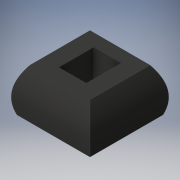
# Autodesk Inventor part: keyswitch-base_cherrymx
Saved by Autodesk Inventor 2016 (Build 200138000, 138)
## iProperties
Created: 2016-12-08
Part Number: keyswitch-base_cherrymx
Material: Generic
Document SubType Name: Modeling
Designer: Cemra JC
Density: 1 g/cm^3
Appearance: Default
Author: Cemra JC
Autodesk Inventor part; units mm, degrees
ref_plane "YZ Plane" through (0, 0, 0) normal (1, 0, 0) x (0, 1, 0)
ref_plane "XZ Plane" through (0, 0, 0) normal (0, 1, 0) x (-1, 0, 0)
ref_plane "XY Plane" through (0, 0, 0) normal (0, 0, 1) x (1, 0, 0)
sketch "Base Loop" plane through (0, 0, 0) normal (0, 1, 0) x (-1, 0, 0)
  line L0 (-7.3, 7.3) -> (7.3, 7.3)
  line L1 (7.3, 7.3) -> (7.3, -7.3)
  line L2 (7.3, -7.3) -> (-7.3, -7.3)
  line L3 (-7.3, -7.3) -> (-7.3, 7.3)
  line L4 (-7.3, 7.3) -> (7.3, -7.3) construction
  line L5 (7.3, 7.3) -> (-7.3, -7.3) construction
  point P0 (0, 0)
  point P1 (0, 0)
  point P2 (0, 0)
  dimension "d0" = 14.6
  dimension "d1" = 14.6
  constraints: 12 end point, 3 midpoint, 2 parallel, 1 coincident, 1 horizontal, 1 perpendicular
  measures "d0" distance of L1.end L2.end
  measures "d1" distance of L0.end L1.end
ref_plane "Mid Plane" through (-7.3, 2, -7.3) normal (0, 1, 0) x (1, 0, 0)
ref_plane "Base Plane" through (-7.3, 0, -7.3) normal (0, 1, 0) x (1, 0, 0)
sketch "Mid Loop" plane through (-7.3, 2, -7.3) normal (0, 1, 0) x (1, 0, 0)
  line L0 (14.5, -14.5) -> (0.1, -14.5)
  line L1 (0.1, -14.5) -> (0.1, -0.1)
  line L2 (0.1, -0.1) -> (14.5, -0.1)
  line L3 (14.5, -0.1) -> (14.5, -14.5)
  line L4 (14.5, -14.5) -> (0.1, -0.1) construction
  line L5 (0.1, -14.5) -> (14.5, -0.1) construction
  point P0 (7.3, -7.3)
  dimension "d3" = 14.4
  dimension "d4" = 14.4
  constraints: 12 end point, 2 midpoint, 2 parallel, 1 horizontal, 1 perpendicular
  measures "d3" distance of L0.end L1.end
  measures "d4" distance of L1.end L2.end
ref_plane "Top Plane" through (-7.3, 8.6, -7.3) normal (0, 1, 0) x (1, 0, 0)
sketch "Top Loop" plane through (-7.3, 8.6, -7.3) normal (0, 1, 0) x (1, 0, 0)
  line L0 (13.3, -13.3) -> (1.3, -13.3)
  line L1 (1.3, -13.3) -> (1.3, -1.3)
  line L2 (1.3, -1.3) -> (13.3, -1.3)
  line L3 (13.3, -1.3) -> (13.3, -13.3)
  line L4 (13.3, -13.3) -> (1.3, -1.3) construction
  line L5 (1.3, -13.3) -> (13.3, -1.3) construction
  point P0 (7.3, -7.3)
  dimension "d6" = 12
  dimension "d7" = 12
  constraints: 12 end point, 2 midpoint, 2 parallel, 1 horizontal, 1 perpendicular
  measures "d6" distance of L1.end L2.end
  measures "d7" distance of L0.end L1.end
loft "Keyswitch Body" add profiles "Base Loop", "Mid Loop", "Top Loop"
sketch "Cut in profile" plane through (-6, 8.6, 6) normal (0, 1, 0) x (1, 0, 0)
  line L0 (8.7, 2.275) -> (3.3, 2.275)
  line L1 (3.3, 2.275) -> (3.3, 9.725)
  line L2 (3.3, 9.725) -> (8.7, 9.725)
  line L3 (8.7, 9.725) -> (8.7, 2.275)
  line L4 (8.7, 2.275) -> (3.3, 9.725) construction
  line L5 (3.3, 2.275) -> (8.7, 9.725) construction
  point P0 (6, 6)
  dimension "d17" = 7.45
  dimension "d18" = 5.4
  constraints: 12 end point, 2 midpoint, 2 parallel, 1 horizontal, 1 perpendicular
  measures "d17" distance of L0.end L1.end
  measures "d18" distance of L0.start L0.end
extrude "Pole Cut in" cut sketch "Cut in profile" against normal blind 6.6
equation "\"d1\" = d0"
equation "\"d3\" = s_bwidth"
equation "\"d4\" = d3"
equation "\"d17\" = s_polebl"
equation "\"d18\" = s_polebw"
equation "\"k_width\" = 18.2"
equation "\"k_height\" = 16.5"
equation "\"k_taper1\" = 1.5"
equation "\"k_taper2\" = 0.5"
equation "\"k_radius\" = 6"
equation "\"k_wthick\" = 1.5"
equation "\"k_ribthick\" = 1.5"
equation "\"k_ribheight\" = 5"
equation "\"k_poleoff\" = 2.275"
equation "\"k_poledia\" = 5.3"
equation "\"k_cmxw\" = 1.55"
equation "\"k_cmxl\" = 4.35"
equation "\"s_bwidth\" = 14.4"
equation "\"s_poleh\" = 3.6"
equation "\"s_polebw\" = 5.4"
equation "\"s_polebl\" = 7.45"
equation "\"b_rshift\" = 50.05"
equation "\"b_ctrl\" = 22.75"
equation "\"b_space\" = 118.3"
equation "\"b_height\" = 77.8"
equation "\"b_width\" = 288"
equation "\"b_lshift\" = 40.95"
equation "\"b_tab\" = 27.3"
equation "\"b_pad\" = 1"
equation "\"b_caps\" = 31.85"
equation "\"k_staper\" = 1"
equation "\"k_ltaper\" = 1.5"
equation "\"k_lradius\" = 6"
equation "\"k_sradius\" = 4"
equation "\"k_height_t\" = 16"
equation "\"k_taper_wide\" = 1.5"
equation "\"k_taper_thin\" = 0.5"
equation "\"k_height_low\" = 15"
equation "\"k_shortening\" = 4.5"
equation "\"k_cmxd\" = 4"
body "Solid1"
